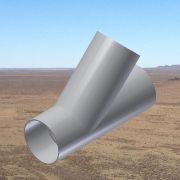
# Autodesk Inventor part: sup-wye
Saved by Autodesk Inventor 2013 SP2 (Build 170200200, 200)
## iProperties
Company: HERA Project
Created: 2013-06-12
Part Number: sup-wye
Material: PVC-Piping
Document SubType Name: Modeling
Designer: David DeBoer
Density: 1.4 g/cm^3
Description: Support PVC wye (could be coupler?)
Mass: 405.128 g
Surface Area: 960.349 cm^2
Volume: 289.377 cm^3
Author: David DeBoer
Title: sup
Autodesk Inventor part; units mm, degrees
ref_plane "YZ Plane" through (0, 0, 0) normal (1, 0, 0) x (0, 1, 0)
ref_plane "XZ Plane" through (0, 0, 0) normal (0, 1, 0) x (-1, 0, 0)
sketch "Sketch1" plane through (0, 0, 0) normal (0, 0, 1) x (1, 0, 0)
  circle A0 centre (0, 0) radius 31.75
  dimension "d0" = 63.5
  constraints: 1 centre point, 1 coincident
  measures "d0" diameter of A0
extrude "Extrusion1" add sketch "Sketch1" along normal blind 174.625
sketch "Sketch2" plane through (0, 0, 174.625) normal (0, 0, 1) x (1, 0, 0)
  circle A0 centre (0, 0) radius 31.75 projected
  circle A1 centre (0, 0) radius 26.2509
  dimension "d3" = 52.5018
  constraints: 1 centre point, 1 coincident
  measures "d3" diameter of A1
extrude "Extrusion2" cut sketch "Sketch2" against normal blind 174.625 contours A1
sketch "Sketch3" plane through (0, 0, 174.625) normal (0, 0, 1) x (1, 0, 0)
  circle A0 centre (0, 0) radius 26.2509 projected
  circle A1 centre (0, 0) radius 31.75 projected
  circle A2 centre (0, 0) radius 30.1625
  dimension "d7" = 60.325
  constraints: 1 centre point, 1 coincident
  measures "d7" diameter of A2
extrude "Extrusion3" cut sketch "Sketch3" against normal blind 38.1 contours A2
sketch "Sketch4" plane through (0, 0, 0) normal (0, 0, -1) x (-1, 0, 0)
  circle A0 centre (0, 0) radius 26.2509 projected
  circle A1 centre (0, 0) radius 31.75 projected
  circle A2 centre (0, 0) radius 30.1625
  dimension "d11" = 60.325
  constraints: 1 centre point, 1 coincident
  measures "d11" diameter of A2
extrude "Extrusion4" cut sketch "Sketch4" against normal blind 38.1 contours A2
sketch "Sketch5" plane through (0, 0, 0) normal (0, 0, -1) x (-1, 0, 0)
  circle A0 centre (0, 0) radius 30.1625 projected
  circle A1 centre (0, 0) radius 31.75 projected
  point P0 (0, 31.75)
  constraints: 1 vertical alignment, 1 other
ref_plane "Work Plane2" through (0, 0, 0) normal (0, 1, 0) x (-1, 0, 0)
ref_plane "Work Plane1" through (0, 31.75, 0) normal (0, 1, 0) x (-1, 0, 0)
sketch "Sketch6" plane through (0, 0, 0) normal (0, 1, 0) x (-1, 0, 0)
  line L0 (-19.7324, 119.8626) -> (17.0407, 119.8626) construction
  line L1 (-30.1625, 174.625) -> (30.1625, 174.625) construction
  point P0 (0, 0)
  dimension "d15" = 54.7624
  constraints: 2 end point, 1 horizontal
  measures "d15" distance between parallel lines of L0 L1
ref_plane "Work Plane3" through (19.7324, 0, 119.8626) normal (0, 0.7071, -0.7071) x (-1, 0, 0)
sketch "Sketch7" plane through (19.7324, 0, 119.8626) normal (0, 0.7071, -0.7071) x (-1, 0, 0)
  circle A0 centre (19.7324, -0.166) radius 31.75
  point P0 (19.7324, -84.7557)
  dimension "d18" = 63.5
  constraints: 1 centre point
  measures "d18" diameter of A0
extrude "Extrusion5" add sketch "Sketch7" along normal blind 119.38
sketch "Sketch8" plane through (0, 84.297, 35.3308) normal (0, 0.7071, -0.7071) x (-1, 0, 0)
  circle A0 centre (0, 0) radius 31.75 projected
  circle A1 centre (0, 0) radius 30.1625
  point P0 (0, -84.5897)
  dimension "d21" = 60.325
  constraints: 1 centre point, 1 coincident
  measures "d21" diameter of A1
extrude "Extrusion6" cut sketch "Sketch8" against normal blind 35.56 contours A1
sketch "Sketch9" plane through (0, 59.1523, 60.4755) normal (0, 0.7071, -0.7071) x (-1, 0, 0)
  circle A0 centre (0, 0) radius 30.1625 projected
  circle A1 centre (0, 0) radius 26.162
  point P0 (0, -84.5897)
  dimension "d24" = 52.324
  constraints: 1 centre point, 1 coincident
  measures "d24" diameter of A1
extrude "Extrusion8" cut sketch "Sketch9" against normal blind 35.56 contours A1
body "Solid1"
